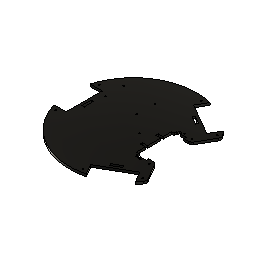
LowerBase v5 (Autodesk Fusion 360 design; units mm, degrees)
Autodesk Fusion 360 part; units mm, degrees
sketch "Sketch1" plane through (0, 0, 0) normal (0, 0, 1) x (1, 0, 0)
  line L0 (-127.0827, 37.5) -> (-102.0827, 37.5)
  line L1 (-102.0827, 37.5) -> (-102.0827, -37.5)
  line L2 (-102.0827, -37.5) -> (-127.0827, -37.5)
  line L3 (0, 0) -> (-132.5, 0) construction
  line L4 (-97.0827, 10) -> (-92.2827, 10)
  line L5 (-92.2827, 10) -> (-92.2827, -10)
  line L6 (-92.2827, -10) -> (-97.0827, -10)
  line L7 (-97.0827, -10) -> (-97.0827, 10)
  arc A0 (-127.0827, 37.5) -> (-132.5, 0) centre (0, 0) ccw construction
  arc A1 (-132.5, 0) -> (-127.0827, -37.5) centre (0, 0) ccw construction
  line L8 (0, 0) -> (66.25, -114.7484) construction
  line L9 (0, 0) -> (66.25, -114.7484) construction
  line L10 (31.0654, -128.8068) -> (18.5654, -107.1562)
  line L11 (18.5654, -107.1562) -> (83.5173, -69.6562)
  line L12 (83.5173, -69.6562) -> (96.0173, -91.3068)
  arc A2 (-127.0827, -37.5) -> (31.0654, -128.8068) centre (0, 0) ccw
  arc A3 (31.0654, -128.8068) -> (66.25, -114.7484) centre (0, 0) ccw construction
  line L13 (37.4811, -84.9191) -> (54.8016, -74.9191)
  line L14 (54.8016, -74.9191) -> (57.2016, -79.076)
  line L15 (57.2016, -79.076) -> (39.8811, -89.076)
  line L16 (39.8811, -89.076) -> (37.4811, -84.9191)
  line L17 (0, 0) -> (132.5, 0) construction
  line L18 (0, 0) -> (66.25, 114.7484) construction
  line L19 (96.0173, 91.3068) -> (83.5173, 69.6562)
  line L20 (83.5173, 69.6562) -> (18.5654, 107.1562)
  line L21 (18.5654, 107.1562) -> (31.0654, 128.8068)
  line L22 (57.2016, 79.076) -> (39.8811, 89.076)
  line L23 (39.8811, 89.076) -> (37.4811, 84.9191)
  line L24 (37.4811, 84.9191) -> (54.8016, 74.9191)
  line L25 (54.8016, 74.9191) -> (57.2016, 79.076)
  circle A4 centre (-115.8879, 45.5) radius 1.5
  circle A5 centre (0, 0) radius 124.5 construction
  circle A6 centre (-115.8879, -45.5) radius 1.5
  circle A7 centre (18.5398, -123.1118) radius 1.5
  circle A8 centre (97.3481, -77.6118) radius 1.5
  circle A9 centre (18.5398, 123.1118) radius 1.5
  line L26 (-102.0827, -18.5) -> (-19.0827, -18.5) construction
  line L27 (-19.0827, -18.5) -> (-19.0827, 18.5) construction
  line L28 (-19.0827, 18.5) -> (-102.0827, 18.5) construction
  line L29 (35.0199, 97.6562) -> (-6.4801, 25.7761) construction
  line L30 (-6.4801, 25.7761) -> (25.5628, 7.2761) construction
  line L31 (25.5628, 7.2761) -> (67.0628, 79.1562) construction
  line L32 (35.0199, -97.6562) -> (-6.4801, -25.7761) construction
  line L33 (-6.4801, -25.7761) -> (25.5628, -7.2761) construction
  line L34 (25.5628, -7.2761) -> (67.0628, -79.1562) construction
  line L35 (-92.0827, 72.5) -> (-21.0827, 72.5) construction
  line L36 (-21.0827, 72.5) -> (-21.0827, 28.5) construction
  line L37 (-21.0827, 28.5) -> (-92.0827, 28.5) construction
  line L38 (-92.0827, 28.5) -> (-92.0827, 72.5) construction
  circle A10 centre (-24.0827, 69.5) radius 1.5
  circle A11 centre (-89.0827, 69.5) radius 1.5
  circle A12 centre (-89.0827, 31.5) radius 1.5
  circle A13 centre (-24.0827, 31.5) radius 1.5
  arc A14 (66.25, -114.7484) -> (96.0173, -91.3068) centre (0, 0) ccw construction
  arc A15 (96.0173, 91.3068) -> (66.25, 114.7484) centre (0, 0) ccw construction
  arc A16 (31.0654, 128.8068) -> (-127.0827, 37.5) centre (0, 0) ccw
  arc A17 (66.25, 114.7484) -> (31.0654, 128.8068) centre (0, 0) ccw construction
  line L39 (125.8662, 41.4) -> (43.6662, 41.4) construction
  line L40 (43.6662, 41.4) -> (43.6662, -41.4) construction
  line L41 (43.6662, -41.4) -> (125.8662, -41.4) construction
  line L42 (43.6662, 13.8) -> (33.1662, 13.8)
  line L43 (33.1662, 13.8) -> (33.1662, 18.6)
  line L44 (33.1662, 18.6) -> (43.6662, 18.6)
  line L45 (68.6662, 36.6) -> (78.2887, 36.6)
  circle A18 centre (97.3481, 77.6118) radius 1.5
  line L46 (104.2763, 73.6118) -> (85.2169, 40.6)
  circle A19 centre (78.2887, 44.6) radius 1.5
  line L47 (43.6662, 13.8) -> (43.6662, -13.8)
  line L48 (43.6662, -13.8) -> (33.1662, -13.8)
  line L49 (33.1662, -13.8) -> (33.1662, -18.6)
  line L50 (33.1662, -18.6) -> (43.6662, -18.6)
  line L51 (68.6662, -36.6) -> (78.2887, -36.6)
  line L52 (104.2763, -73.6118) -> (85.2169, -40.6)
  circle A20 centre (78.2887, -44.6) radius 1.5
  arc A21 (132.5, 0) -> (125.8662, 41.4) centre (0, 0) ccw construction
  arc A22 (103.6034, 82.599) -> (96.0173, 91.3068) centre (0, 0) ccw
  arc A23 (106.9418, 78.2286) -> (103.6034, 82.599) centre (0, 0) ccw construction
  line L53 (106.9418, 78.2286) -> (104.2763, 73.6118) construction
  arc A24 (125.8662, 41.4) -> (106.9418, 78.2286) centre (0, 0) ccw construction
  line L54 (78.2887, 36.6) -> (82.9075, 36.6) construction
  arc A25 (85.2169, 40.6) -> (78.2887, 36.6) centre (78.2887, 44.6) ccw construction
  arc A26 (78.2887, 36.6) -> (85.2169, 40.6) centre (78.2887, 44.6) ccw
  line L55 (85.2169, 40.6) -> (82.9075, 36.6) construction
  line L56 (78.2887, -36.6) -> (82.9075, -36.6) construction
  line L57 (85.2169, -40.6) -> (82.9075, -36.6) construction
  arc A27 (78.2887, -36.6) -> (85.2169, -40.6) centre (78.2887, -44.6) ccw construction
  arc A28 (85.2169, -40.6) -> (78.2887, -36.6) centre (78.2887, -44.6) ccw
  arc A29 (96.0173, -91.3068) -> (103.6034, -82.599) centre (0, 0) ccw
  arc A30 (125.8662, -41.4) -> (132.5, 0) centre (0, 0) ccw construction
  arc A31 (106.9418, -78.2286) -> (125.8662, -41.4) centre (0, 0) ccw construction
  line L58 (106.9418, -78.2286) -> (104.2763, -73.6118) construction
  arc A32 (103.6034, -82.599) -> (106.9418, -78.2286) centre (0, 0) ccw construction
  arc A33 (104.2763, -73.6118) -> (103.6034, -82.599) centre (97.3481, -77.6118) ccw construction
  arc A34 (103.6034, -82.599) -> (104.2763, -73.6118) centre (97.3481, -77.6118) ccw
  arc A35 (103.6034, 82.599) -> (104.2763, 73.6118) centre (97.3481, 77.6118) ccw construction
  arc A36 (104.2763, 73.6118) -> (103.6034, 82.599) centre (97.3481, 77.6118) ccw
  line L59 (33.1662, 13.8) -> (33.1662, -13.8) construction
  line L60 (48.6662, 41.4) -> (48.6662, 36.6)
  line L61 (68.6662, 41.4) -> (68.6662, 36.6)
  line L62 (48.6662, 36.6) -> (43.6662, 36.6)
  line L63 (43.6662, 18.6) -> (43.6662, 36.6)
  line L64 (50.6662, 41.4) -> (50.6662, 45.4)
  line L65 (50.6662, 45.4) -> (56.6662, 45.4)
  line L66 (56.6662, 45.4) -> (56.6662, 41.4)
  circle A37 centre (60.6662, 46.4) radius 1.5
  line L67 (48.6662, 41.4) -> (50.6662, 41.4)
  line L68 (56.6662, 41.4) -> (68.6662, 41.4)
  line L69 (43.6662, -36.6) -> (48.6662, -36.6)
  line L70 (48.6662, -36.6) -> (48.6662, -41.4)
  line L71 (48.6662, -41.4) -> (50.6662, -41.4)
  line L72 (50.6662, -41.4) -> (50.6662, -45.4)
  line L73 (50.6662, -45.4) -> (56.6662, -45.4)
  line L74 (56.6662, -45.4) -> (56.6662, -41.4)
  line L75 (56.6662, -41.4) -> (68.6662, -41.4)
  line L76 (68.6662, -41.4) -> (68.6662, -36.6)
  line L77 (43.6662, -18.6) -> (43.6662, -36.6)
  circle A38 centre (60.6662, -46.4) radius 1.5
  circle A39 centre (12.9173, 0) radius 1.5
  point P0 (-102.0827, 0)
  point P1 (-97.0827, 0)
  point P2 (51.0413, -88.4062)
  point P3 (48.5413, -84.076)
  point P4 (51.0413, 88.4062)
  point P5 (48.5413, 84.076)
  point P6 (-19.0827, 0)
  point P7 (9.5413, 16.5261)
  point P8 (9.5413, -16.5261)
  point P9 (43.6662, 0)
  point P10 (53.6662, 45.4)
  point P11 (53.6662, -45.4)
  point P12 (12.9173, 0)
  dimension "d1" = 265
  dimension "d2" = 75
  dimension "d3" = 25
  dimension "d4" = 4.8
  dimension "d5" = 20
  dimension "d6" = 5
  dimension "d17" = 120
  dimension "d19" = 132.5
  dimension "d20" = 75
  dimension "d21" = 25
  dimension "d22" = 20
  dimension "d23" = 4.8
  dimension "d24" = 5
  dimension "d25" = 132.5
  dimension "d28" = 60
  dimension "d29" = 75
  dimension "d30" = 25
  dimension "d31" = 4.8
  dimension "d32" = 20
  dimension "d33" = 5
  dimension "d34" = 3
  dimension "d35" = 8
  dimension "d36" = 249
  dimension "d37" = 3
  dimension "d38" = 8
  dimension "d39" = 3
  dimension "d40" = 8
  dimension "d41" = 3
  dimension "d42" = 8
  dimension "d49" = 3
  dimension "d50" = 8
  dimension "d53" = 37
  dimension "d55" = 37
  dimension "d57" = 78
  dimension "d58" = 78
  dimension "d59" = 37
  dimension "d60" = 78
  dimension "d61" = 71
  dimension "d62" = 44
  dimension "d63" = 10
  dimension "d64" = 10
  dimension "d75" = 3
  dimension "d76" = 3
  dimension "d77" = 3
  dimension "d78" = 3
  dimension "d85" = 3
  dimension "d86" = 3
  dimension "d87" = 3
  dimension "d88" = 3
  dimension "d89" = 3
  dimension "d90" = 3
  dimension "d91" = 3
  dimension "d92" = 3
  dimension "d156" = 82.8
  dimension "d157" = 82.2
  dimension "d161" = 4.8
  dimension "d162" = 13.8
  dimension "d167" = 3
  dimension "d168" = 8
  dimension "d169" = 8
  dimension "d170" = 3
  dimension "d171" = 8
  dimension "d172" = 8
  dimension "d173" = 10.5
  dimension "d174" = 4.8
  dimension "d175" = 27.6
  dimension "d180" = 8
  dimension "d181" = 3
  dimension "d182" = 8
  dimension "d183" = 8
  dimension "d184" = 4.8
  dimension "d185" = 4.8
  dimension "d186" = 20
  dimension "d187" = 5
  dimension "d188" = 4
  dimension "d189" = 6
  dimension "d190" = 10
  dimension "d191" = 3
  dimension "d193" = 17
  dimension "d194" = 5
  dimension "d195" = 4.8
  dimension "d196" = 5
  dimension "d197" = 6
  dimension "d198" = 4
  dimension "d199" = 10
  dimension "d200" = 20
  dimension "d201" = 3
  dimension "d202" = 5
  dimension "d203" = 17
  dimension "d204" = 4.8
  dimension "d205" = 115
  dimension "d206" = 3
  constraint coincident L3.start A0.centre
  constraint horizontal L0
  constraint perpendicular L0 L1
  constraint horizontal L2
  constraint perpendicular L1 L3
  constraint midpoint L1 P0
  constraint coincident L3 P0
  constraint horizontal L4
  constraint vertical L5
  constraint horizontal L6
  constraint vertical L7
  constraint midpoint L7 P1
  constraint coincident L3 P1
  constraint concentric A0 A2
  constraint concentric A1 A2
  constraint coincident L8.end A2
  constraint parallel L8 L10
  constraint perpendicular L8 L11
  constraint coincident L12.end A2
  constraint perpendicular L11 L12
  constraint midpoint L11 P2
  constraint coincident L8 P2
  constraint concentric A2 A3
  constraint perpendicular L12 L13
  constraint perpendicular L13 L14
  constraint perpendicular L9 L15
  constraint parallel L8 L16
  constraint midpoint L15 P3
  constraint coincident L8 P3
  constraint horizontal L17
  constraint parallel L18 L19
  constraint perpendicular L18 L20
  constraint perpendicular L20 L21
  constraint midpoint L20 P4
  constraint coincident L18 P4
  constraint perpendicular L18 L22
  constraint perpendicular L22 L23
  constraint perpendicular L18 L24
  constraint parallel L18 L25
  constraint midpoint L22 P5
  constraint coincident L18 P5
  constraint coincident A4.centre A5
  constraint coincident A5 A6.centre
  constraint coincident A5 A7.centre
  constraint coincident A5 A8.centre
  constraint coincident A5 A9.centre
  constraint coincident L1 L26.start
  constraint perpendicular L1 L26
  constraint perpendicular L3 L27
  constraint coincident L1 L28.end
  constraint perpendicular L1 L28
  constraint midpoint L27 P6
  constraint coincident L3 P6
  constraint coincident L20 L29.start
  constraint perpendicular L20 L29
  constraint perpendicular L18 L30
  constraint coincident L20 L31.end
  constraint perpendicular L20 L31
  constraint midpoint L30 P7
  constraint coincident L18 P7
  constraint coincident L11 L32.start
  constraint perpendicular L11 L32
  constraint perpendicular L32 L33
  constraint coincident L11 L34.end
  constraint perpendicular L11 L34
  constraint midpoint L33 P8
  constraint coincident L8 P8
  constraint horizontal L35
  constraint vertical L36
  constraint horizontal L37
  constraint vertical L38
  constraint coincident L17.end A14
  constraint concentric A14 A15
  constraint concentric A14 A29
  constraint concentric A15 A21
  constraint concentric A15 A16
  constraint concentric A15 A17
  constraint horizontal L39
  constraint coincident L41.end A29
  constraint perpendicular L40 L41
  constraint midpoint L40 P9
  constraint coincident L17 P9
  constraint coincident L40 L42.start
  constraint perpendicular L40 L42
  constraint perpendicular L42 L43
  constraint coincident L40 L44.end
  constraint perpendicular L40 L44
  constraint coincident A5 A18.centre
  constraint parallel L18 L46
  constraint coincident L40 L47.end
  constraint perpendicular L40 L48
  constraint perpendicular L48 L49
  constraint coincident L40 L50.end
  constraint perpendicular L40 L50
  constraint parallel L8 L52
  constraint concentric A8 A33
  constraint tangent L52 A33
  constraint concentric A20 A27
  constraint tangent L51 A27
  constraint concentric A19 A25
  constraint tangent L45 A25
  constraint concentric A18 A35
  constraint tangent L46 A35
  constraint concentric A21 A22
  constraint concentric A21 A23
  constraint tangent L53 A35
  constraint concentric A21 A24
  constraint tangent L54 A25
  constraint concentric A25 A26
  constraint tangent L55 A35
  constraint tangent L56 A27
  constraint tangent L57 A33
  constraint concentric A27 A28
  constraint concentric A29 A30
  constraint concentric A29 A31
  constraint tangent L58 A33
  constraint concentric A29 A32
  constraint concentric A33 A34
  constraint concentric A35 A36
  constraint perpendicular L48 L59
  constraint perpendicular L39 L63
  constraint coincident L39 L60.start
  constraint coincident L39 L61.start
  constraint perpendicular L39 L60
  constraint coincident L40 L62.end
  constraint perpendicular L62 L63
  constraint perpendicular L45 L61
  constraint perpendicular L64 L65
  constraint midpoint L65 P10
  constraint perpendicular L64 L67
  constraint perpendicular L61 L68
  constraint perpendicular L65 L66
  constraint perpendicular L39 L66
  constraint coincident L40 L69.start
  constraint perpendicular L40 L69
  constraint coincident L41 L70.end
  constraint perpendicular L41 L70
  constraint coincident L41 L71.end
  constraint perpendicular L41 L72
  constraint perpendicular L70 L73
  constraint coincident L41 L74.end
  constraint perpendicular L41 L74
  constraint coincident L41 L75.end
  constraint perpendicular L41 L76
  constraint midpoint L73 P11
  constraint perpendicular L51 L76
  constraint coincident L17 P12
  constraint coincident P12 A39.centre
  measures "d1" diameter of A2
  measures "d2" distance of L0.end L1.end
  measures "d3" distance of L1.end L2.end
  measures "d4" distance of L4.start L4.end
  measures "d5" distance of L4.end L5.end
  measures "d6" distance of L1 L7
  measures "d17" angle of L3 L8
  measures "d19" distance of L3.start L8.end
  measures "d20" distance of L10.end L11.end
  measures "d21" distance of L10.start L10.end
  measures "d22" distance of L13.start L13.end
  measures "d23" distance of L13.start L15.end
  measures "d24" distance of L11 L15
  measures "d25" distance of L3.start L17.end
  measures "d28" angle of L17 L18
  measures "d29" distance of L19.end L20.end
  measures "d30" distance of L19.start L19.end
  measures "d31" distance of L22.start L24.end
  measures "d32" distance of L23.end L24.end
  measures "d33" distance of L20 L22
  measures "d34" diameter of A4
  measures "d35" distance of L0 A4.centre
  measures "d36" diameter of A5
  measures "d37" diameter of A6
  measures "d38" distance of L2 A6.centre
  measures "d39" diameter of A7
  measures "d40" distance of L10 A7.centre
  measures "d41" diameter of A8
  measures "d42" distance of L12 A8.centre
  measures "d49" diameter of A9
  measures "d50" distance of L21 A9.centre
  measures "d53" distance of L26.end L27.end
  measures "d55" distance of L29.end L30.end
  measures "d57" distance of L7 L27
  measures "d58" distance of L22 L30
  measures "d59" distance of L32.end L33.end
  measures "d60" distance of L15 L33
  measures "d61" distance of L35.start L35.end
  measures "d62" distance of L35.start L37.end
  measures "d63" distance of L28 L37
  measures "d64" distance of L1 L38
  measures "d75" diameter of A10
  measures "d76" diameter of A11
  measures "d77" diameter of A12
  measures "d78" diameter of A13
  measures "d85" distance of L37 A13.centre
  measures "d86" distance of L36 A13.centre
  measures "d87" distance of L36 A10.centre
  measures "d88" distance of L35 A10.centre
  measures "d89" distance of L35 A11.centre
  measures "d90" distance of L38 A11.centre
  measures "d91" distance of L38 A12.centre
  measures "d92" distance of L37 A12.centre
  measures "d156" distance of L39.end L40.end
  measures "d157" distance of L39.start L39.end
  measures "d161" distance of L42.end L43.end
  measures "d162" distance of P9 L42
  measures "d167" diameter of A18
  measures "d168" distance of L19 A18.centre
  measures "d169" distance of A18.centre L46
  measures "d170" diameter of A19
  measures "d171" distance of L46 A19.centre
  measures "d172" distance of L45 A19.centre
  measures "d173" distance of L47.end L48.end
  measures "d174" distance of L48.end L49.end
  measures "d175" distance of L42 L48
  measures "d180" distance of A8.centre L52
  measures "d181" diameter of A20
  measures "d182" distance of L52 A20.centre
  measures "d183" distance of L51 A20.centre
  measures "d184" distance of L60.start L60.end
  measures "d185" distance of L61.start L45.start
  measures "d186" distance of L60 L61
  measures "d187" distance of L60.end L62.end
  measures "d188" distance of L64.start L64.end
  measures "d189" distance of L64.end L65.end
  measures "d190" distance of L40 P10
  measures "d191" diameter of A37
  measures "d193" distance of L40 A37.centre
  measures "d194" distance of L39 A37.centre
  measures "d195" distance of L41 L69
  measures "d196" distance of L69.start L69.end
  measures "d197" distance of L72.end L73.end
  measures "d198" distance of L71.end L72.end
  measures "d199" distance of L40 P11
  measures "d200" distance of L70 L76
  measures "d201" diameter of A38
  measures "d202" distance of L75 A38.centre
  measures "d203" distance of L40 A38.centre
  measures "d204" distance of L75.end L51.start
  measures "d205" distance of L1 P12
  measures "d206" diameter of A39
extrude "Extrude1" add sketch "Sketch1" against normal blind 4.8
